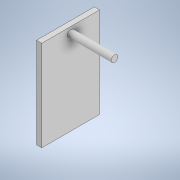
# Autodesk Inventor part: sample-transfer_slider
Saved by Autodesk Inventor 2020 (Build 240168000, 168)
## iProperties
Created: 2019-08-28
Part Number: sample-transfer_slider
Material: Generic
Document SubType Name: Modeling
Designer: rainer
Density: 1 g/cm^3
Appearance: Default
Author: rainer
Autodesk Inventor part; units mm, degrees
ref_plane "YZ Plane" through (0, 0, 0) normal (1, 0, 0) x (0, 1, 0)
ref_plane "XZ Plane" through (0, 0, 0) normal (0, 1, 0) x (-1, 0, 0)
ref_plane "XY Plane" through (0, 0, 0) normal (0, 0, 1) x (1, 0, 0)
sketch "Sketch1" plane through (0, 0, 0) normal (1, 0, 0) x (0, 1, 0)
  line L0 (20, 9.9) -> (-20, 9.9)
  line L1 (-20, 9.9) -> (-20, -9.9)
  line L2 (-20, -9.9) -> (20, -9.9)
  line L3 (20, -9.9) -> (20, 9.9)
  point P0 (0, 0)
  point P1 (0, 9.9)
  point P2 (-20, 0)
  dimension "d0" = 19.8
  dimension "d1" = 40
  constraints: 8 end point, 2 midpoint, 2 parallel, 1 horizontal, 1 horizontal alignment, 1 perpendicular, 1 vertical alignment
  measures "d0" distance of L0.end L1.end
  measures "d1" distance of L1.end L2.end
extrude "Extrusion1" add sketch "Sketch1" along normal blind 1.8
sketch "Sketch2" plane through (1.8, 0, 0) normal (1, 0, 0) x (0, 0, -1)
  circle A0 centre (0, 14) radius 1.15
  line L0 (-9.9, -20) -> (9.9, -20) projected
  point P0 (0, 0)
  dimension "d4" = 2.3
  dimension "d5" = 34
  constraints: 1 centre point
  measures "d4" diameter of A0
  measures "d5" distance from line of L0 A0.centre
extrude "Extrusion2" add sketch "Sketch2" along normal blind 10
thicken "Thicken1" operation add thickness 10 both sides no extend neighbours yes toward (0, 1, 0) faces at (0.6, -20, 3.3)
thicken "Thicken2" operation add thickness 5 both sides no extend neighbours yes toward (0, -1, 0) faces at (0.6, -10, 3.3)
thicken "Thicken3" operation add thickness 2 both sides no extend neighbours yes toward (0, 1, 0) faces at (0.6, -15, 3.3)
thicken "Thicken4" operation add thickness 4 both sides no extend neighbours yes toward (0, -1, 0) faces at (0.6, 20, -3.3)
thicken "Thicken5" operation add thickness 2 both sides no extend neighbours yes toward (0, -1, 0) faces at (0.6, -13, 3.3)
thicken "Thicken6" operation add thickness 5 both sides no extend neighbours yes toward (1, 0, 0) faces at (11.8, 13.5623, 0.2869)
body "Solid1"
